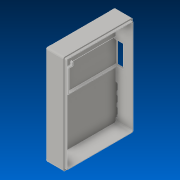
# Autodesk Inventor part: Bottom
Saved by Autodesk Inventor 2016 (Build 200138000, 138)
## iProperties
Created: 2015-08-21
Part Number: Bottom
Material: Generic
Document SubType Name: Modeling
Designer: Moffitt
Density: 1 g/cm^3
Appearance: Default
Author: Moffitt
Autodesk Inventor part; units mm, degrees
ref_plane "YZ Plane" through (0, 0, 0) normal (1, 0, 0) x (0, 1, 0)
ref_plane "XZ Plane" through (0, 0, 0) normal (0, 1, 0) x (-1, 0, 0)
ref_plane "XY Plane" through (0, 0, 0) normal (0, 0, 1) x (1, 0, 0)
sketch "Very Bottom" plane through (0, 0, 0) normal (1, 0, 0) x (0, 1, 0)
  line L0 (98.706, 61.2459) -> (-101.294, 61.2459)
  line L1 (-101.294, 61.2459) -> (-101.294, -78.7541)
  line L2 (-101.294, -78.7541) -> (98.706, -78.7541)
  line L3 (98.706, -78.7541) -> (98.706, 61.2459)
  point P0 (0, 0)
  dimension "d4" = 140
  dimension "d5" = 200
  constraints: 8 end point, 2 parallel, 1 horizontal, 1 perpendicular
  measures "d4" distance of L2.end L0.start
  measures "d5" distance of L1.end L2.end
extrude "Extrusion1" add sketch "Very Bottom" along normal blind 6
sketch "Walls A" plane through (6, 0, 0) normal (1, 0, 0) x (0, 0, -1)
  line L0 (-57.2459, 94.706) -> (74.7541, 94.706)
  line L1 (74.7541, 94.706) -> (74.7541, -97.294)
  line L2 (74.7541, -97.294) -> (-57.2459, -97.294)
  line L3 (-57.2459, -97.294) -> (-57.2459, 94.706)
  line L4 (78.7541, 98.706) -> (-61.2459, 98.706) projected
  line L5 (-61.2459, -101.294) -> (78.7541, -101.294) projected
  line L6 (-61.2459, 98.706) -> (-61.2459, -101.294) projected
  line L7 (78.7541, -101.294) -> (78.7541, 98.706) projected
  point P0 (0, 0)
  dimension "d6" = 4
  dimension "d7" = 4
  dimension "d8" = 4
  dimension "d9" = 4
  constraints: 8 end point, 2 parallel, 1 horizontal, 1 perpendicular
  measures "d6" distance between parallel lines of L4 L0
  measures "d7" distance between parallel lines of L5 L2
  measures "d8" distance between parallel lines of L3 L6
  measures "d9" distance between parallel lines of L7 L1
extrude "Walls" add sketch "Walls A" along normal blind 34
sketch "Back Panel" plane through (0, -101.294, -78.7541) normal (0, 0, -1) x (-1, 0, 0)
  line L0 (0, 0) -> (-40, 0) projected
  line L1 (-6, 4) -> (-6, 196) projected
  line L2 (-6, 103.5669) -> (-21, 103.5669)
  line L3 (-21, 103.5669) -> (-21, 147.5669)
  line L4 (-21, 147.5669) -> (-6, 147.5669)
  line L5 (-6, 147.5669) -> (-6, 103.5669)
  line L6 (-6, 147.5669) -> (-2, 147.5669)
  line L7 (-2, 147.5669) -> (-2, 103.5669)
  line L8 (-2, 103.5669) -> (-6, 103.5669)
  line L9 (-6, 103.5669) -> (-6, 147.5669)
  point P0 (0, 101.294)
  dimension "d33" = 44
  dimension "d34" = 15
  dimension "d52" = 4
  constraints: 16 end point, 4 parallel, 2 horizontal, 2 perpendicular, 1 point on line
  measures "d33" distance of L2.end L3.end
  measures "d34" distance of L3.end L4.end
  measures "d52" distance of L4.end L6.end
fillet "Fillet1" radius 3 12 edges at (20, 98.706, -78.7541) (0, -1.294, -78.7541) (20, -101.294, -78.7541) (0, -101.294, -8.7541) (20, -101.294, 61.2459) (0, -1.294, 61.2459) (20, 98.706, 61.2459) (23, 94.706, 57.2459) (23, 94.706, -74.7541) (23, -97.294, -74.7541) (23, -97.294, 57.2459) (0, 98.706, -8.7541)
sketch "Sketch5" plane through (6, 0, 0) normal (1, 0, 0) x (0, 0, -1)
  line L0 (77.7541, 2.273) -> (70.7541, 2.273) projected
  line L1 (77.7541, 2.273) -> (-22.2459, 2.273)
  line L2 (-22.2459, 2.273) -> (-22.2459, 46.273)
  line L3 (-22.2459, 46.273) -> (77.7541, 46.273)
  line L4 (77.7541, 46.273) -> (77.7541, 2.273)
  line L5 (74.7541, 91.706) -> (74.7541, -94.294) projected
  line L6 (-14.2459, 46.273) -> (74.7541, 46.273)
  line L7 (74.7541, 46.273) -> (74.7541, 50.273)
  line L8 (74.7541, 50.273) -> (-14.2459, 50.273)
  line L9 (-14.2459, 50.273) -> (-14.2459, 46.273)
  point P0 (0, 0)
  dimension "d43" = 100
  dimension "d47" = 8
  dimension "d48" = 4
  constraints: 16 end point, 4 parallel, 2 horizontal, 2 perpendicular, 1 point on line, 2 other
  measures "d43" distance of L2.end L3.end
  measures "d47" distance from line of L2.end L9
  measures "d48" distance of L8.end L6.start
extrude "PCB Slot" cut sketch "Sketch5" against normal blind 2.5
sketch "Sketch9" plane through (3, 98.706, -75.7541) normal (0, 1, 0) x (1, 0, 0)
  line L0 (-3, 0) -> (-3, -134) projected
  line L1 (-3, -132.5) -> (-1.5, -132.5)
  line L2 (-1.5, -132.5) -> (-1.5, -130.5)
  line L3 (-1.5, -130.5) -> (-3, -130.5)
  line L4 (-3, -130.5) -> (-3, -132.5)
  line L5 (-3, -128.5) -> (-1.5, -128.5)
  line L6 (-1.5, -128.5) -> (-1.5, -126.5)
  line L7 (-1.5, -126.5) -> (-3, -126.5)
  line L8 (-3, -126.5) -> (-3, -128.5)
  line L9 (-3, -1.5) -> (-1.5, -1.5)
  line L10 (-1.5, -1.5) -> (-1.5, -3.5)
  line L11 (-1.5, -3.5) -> (-3, -3.5)
  line L12 (-3, -3.5) -> (-3, -1.5)
  line L13 (-3, -5.5) -> (-1.5, -5.5)
  line L14 (-1.5, -5.5) -> (-1.5, -7.5)
  line L15 (-1.5, -7.5) -> (-3, -7.5)
  line L16 (-3, -7.5) -> (-3, -5.5)
  point P0 (-3, -75.7541)
  dimension "d66" = 1.5
  dimension "d67" = 1.5
  dimension "d68" = 2
  dimension "d69" = 2
  dimension "d70" = 2
  dimension "d71" = 2
  dimension "d72" = 2
  dimension "d73" = 1.5
  dimension "d74" = 2
  dimension "d75" = 1.5
  dimension "d76" = 1.5
  constraints: 32 end point, 8 parallel, 5 point on line, 4 horizontal, 4 perpendicular
  measures "d66" distance of L14.end L15.end
  measures "d67" distance of L10.end L11.end
  measures "d68" distance of L9.end L10.end
  measures "d69" distance of L13.end L14.end
  measures "d70" distance between parallel lines of L11 L13
  measures "d71" distance of L1.end L2.end
  measures "d72" distance of L5.end L6.end
  measures "d73" distance from line of L0.end L1
  measures "d74" distance between parallel lines of L5 L3
  measures "d75" distance of L6.end L7.end
  measures "d76" distance from line of L0.start L9
extrude "Extrusion8" cut sketch "Sketch9" against normal blind 200
extrude "Extrusion9" cut sketch "Back Panel" against normal blind 5 contours L2 L3 L4 L1
chamfer "Chamfer4" distance 2 angle 45 1 edges at (6, 50.273, -30.2541)
sketch "Sketch10" plane through (6, 0, 0) normal (1, 0, 0) x (0, 0, -1)
  line L0 (74.7541, 52.273) -> (74.7541, 91.706) projected
  line L1 (-16.2459, 54.4026) -> (-16.2459, 48.273)
  line L2 (-16.2459, 48.273) -> (-24.2459, 48.273)
  line L3 (-24.2459, 48.273) -> (-24.2459, 0.273)
  line L4 (-24.2459, 0.273) -> (74.7541, 0.273)
  line L5 (74.7541, 91.706) -> (74.7541, -94.294) projected
  line L6 (74.7541, 46.273) -> (74.7541, 2.273) projected
  line L7 (74.7541, 2.273) -> (-22.2459, 2.273)
  line L8 (-22.2459, 2.273) -> (-22.2459, 46.273) projected
  line L9 (-22.2459, 2.273) -> (-22.2459, 46.273)
  line L10 (-22.2459, 46.273) -> (-14.2459, 46.273) projected
  line L11 (-22.2459, 46.273) -> (-14.2459, 46.273)
  line L12 (74.7541, 52.273) -> (-14.2459, 52.273) projected
  line L13 (-14.2459, 46.273) -> (-14.2459, 52.273)
  line L14 (-14.2459, 52.273) -> (-14.2459, 54.4026)
  line L15 (-14.2459, 54.4026) -> (-16.2459, 54.4026)
  line L16 (71.7541, 2.273) -> (71.7541, -94.294) projected
  line L17 (71.7541, 2.273) -> (74.7541, 2.273)
  line L18 (77.7541, 2.273) -> (-22.2459, 2.273) projected
  line L19 (74.7541, 0.273) -> (71.7541, 0.273)
  point P0 (0, 0)
  point P1 (71.7541, 52.273)
  dimension "d84" = 2
  dimension "d85" = 2
  dimension "d86" = 2
  dimension "d87" = 2
  constraints: 24 end point, 5 perpendicular, 4 point on line, 2 collinear, 2 horizontal
  measures "d84" distance between parallel lines of L13 L1
  measures "d85" distance between parallel lines of L11 L2
  measures "d86" distance between parallel lines of L8 L3
  measures "d87" distance between parallel lines of L4 L7
extrude "Extrusion10" add sketch "Sketch10" along normal blind 3 contours L15 L14 L13 L10 L8 L7 L16 L4 L3 L2 L1 | L16 L7 L5 L4
fillet "Fillet5" radius 1 18 edges at (6, 54.4026, 15.2459) (6, 51.3378, 16.2459) (6, 48.273, 20.2459) (6, 24.273, 24.2459) (6, 0.273, -25.2541) (9, 0.273, -25.2541) (9, 24.273, 24.2459) (7.5, 0.273, 24.2459) (7.5, 48.273, 24.2459) (9, 48.273, 20.2459) (9, 51.3378, 16.2459) (9, 54.4026, 15.2459) (7.5, 54.4026, 16.2459) (7.5, 48.273, 16.2459) (6, 52.273, -30.2541) (6.25, 46.273, 14.2459) (12.25, 46.273, -74.7541) (15, 2.273, -74.7541)
sketch "Sketch11" plane through (40, 95.706, -78.7541) normal (0, 0, -1) x (-1, 0, 0)
  line L0 (34, -96.4331) -> (34, -190) projected
  line L1 (34, -181.567) -> (30, -181.567)
  line L2 (30, -181.567) -> (30, -167.567)
  line L3 (30, -167.567) -> (34, -167.567)
  line L4 (34, -167.567) -> (34, -181.567)
  line L5 (30, -160.567) -> (34, -160.567)
  line L6 (34, -160.567) -> (34, -146.567)
  line L7 (34, -146.567) -> (30, -146.567)
  line L8 (30, -146.567) -> (30, -160.567)
  line L9 (30, -139.567) -> (34, -139.567)
  line L10 (34, -139.567) -> (34, -125.567)
  line L11 (34, -125.567) -> (30, -125.567)
  line L12 (30, -125.567) -> (30, -139.567)
  point P0 (40, -95.706)
  dimension "d91" = 14
  dimension "d92" = 4
  dimension "d93" = 7
  dimension "d94" = 14
  dimension "d95" = 4
  dimension "d96" = 7
  dimension "d97" = 14
  dimension "d98" = 4
  constraints: 24 end point, 6 parallel, 3 horizontal, 3 perpendicular, 3 point on line
  measures "d91" distance between parallel lines of L3 L1
  measures "d92" distance of L1.start L1.end
  measures "d93" distance between parallel lines of L5 L3
  measures "d94" distance of L7.end L5.start
  measures "d95" distance of L6.end L7.end
  measures "d96" distance between parallel lines of L9 L7
  measures "d97" distance of L11.end L9.start
  measures "d98" distance of L10.end L11.end
extrude "Extrusion11" cut sketch "Sketch11" against normal blind 5
sketch "Sketch13" plane through (40, -94.294, -74.7541) normal (0, 0, 1) x (1, 0, 0)
  line L0 (-34, 0) -> (-34, 186) projected
  line L1 (-30, 4.933) -> (-34, 4.933)
  line L2 (-34, 4.933) -> (-34, 67.933)
  line L3 (-34, 67.933) -> (-30, 67.933)
  line L4 (-30, 67.933) -> (-30, 4.933)
  line L5 (-34, 8.433) -> (-30, 8.433) projected
  line L6 (-30, 64.433) -> (-34, 64.433) projected
  line L7 (-30, 29.433) -> (-30, 43.433) projected
  point P0 (-40, 94.294)
  dimension "d103" = 3.5
  dimension "d104" = 3.5
  dimension "d105" = 0
  constraints: 8 end point, 2 parallel, 1 horizontal, 1 perpendicular, 1 point on line
  measures "d103" distance between parallel lines of L5 L1
  measures "d104" distance between parallel lines of L3 L6
  measures "d105" distance between parallel lines of L7 L4
extrude "Extrusion12" cut sketch "Sketch13" against normal blind 2
chamfer "Chamfer5" distance 4 angle 10 3 edges at (10, -78.861, -78.7541) (10, -57.861, -78.7541) (10, -36.861, -78.7541) measured on face at (10.5, -36.861, -78.7541) measured on face at (10.5, -57.861, -78.7541) measured on face at (10.5, -78.861, -78.7541)
sketch "Sketch14" plane through (40, 0, 0) normal (1, 0, 0) x (0, 0, -1)
  line L0 (73.7541, 95.706) -> (-56.2459, 95.706)
  line L1 (-58.2459, 93.706) -> (-58.2459, -96.294)
  line L2 (-56.2459, -98.294) -> (73.7541, -98.294)
  line L3 (75.7541, -96.294) -> (75.7541, 93.706)
  line L4 (75.7541, 98.706) -> (-58.2459, 98.706) projected
  line L5 (74.7541, 91.706) -> (74.7541, -94.294) projected
  line L6 (71.7541, -97.294) -> (-54.2459, -97.294) projected
  line L7 (-61.2459, 95.706) -> (-61.2459, -98.294) projected
  arc A0 (75.7541, 93.706) -> (73.7541, 95.706) centre (73.7541, 93.706) ccw
  arc A1 (73.7541, -98.294) -> (75.7541, -96.294) centre (73.7541, -96.294) ccw
  arc A2 (-58.2459, -96.294) -> (-56.2459, -98.294) centre (-56.2459, -96.294) ccw
  line L8 (78.7541, 98.706) -> (-61.2459, 98.706)
  line L9 (-61.2459, 98.706) -> (-61.2459, -99.294)
  line L10 (-59.2459, -101.294) -> (78.7541, -101.294)
  line L11 (78.7541, -101.294) -> (78.7541, 98.706)
  arc A3 (-61.2459, -99.294) -> (-59.2459, -101.294) centre (-59.2459, -99.294) ccw
  line L12 (-58.2459, -101.294) -> (75.7541, -101.294) projected
  arc A4 (-56.2459, 95.706) -> (-58.2459, 93.706) centre (-56.2459, 93.706) ccw
  point P0 (0, 0)
  point P1 (-58.2459, 95.706)
  dimension "d111" = 3
  dimension "d112" = 1
  dimension "d113" = 1
  dimension "d114" = 3
  dimension "d115" = 2
  dimension "d116" = 2
  dimension "d117" = 0
  dimension "d120" = 2
  constraints: 16 end point, 10 point on circle, 10 tangent, 5 centre point, 4 parallel, 2 equal radius, 2 horizontal, 2 perpendicular, 2 point on line
  measures "d111" distance between parallel lines of L4 L0
  measures "d112" distance between parallel lines of L5 L3
  measures "d113" distance between parallel lines of L6 L2
  measures "d114" distance between parallel lines of L7 L1
  measures "d115" radius of A0
  measures "d116" radius of A3
  measures "d117" distance between parallel lines of L10 L12
  measures "d120" radius of A4
extrude "Extrusion13" cut sketch "Sketch14" against normal blind 4
body "Solid1"
